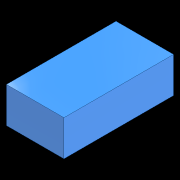
# Autodesk Inventor part: 2s 250mAh Mockup
Saved by Autodesk Inventor 2022 (Build 260153000, 153)
## iProperties
Created: 2022-09-18
Part Number: 2s 250mAh Mockup
Material: Generic
Document SubType Name: Modeling
Designer: tandu
Density: 1.4652 g/cm^3
Appearance: Cyan
Mass: 16 g
Surface Area: 32.66 cm^2
Volume: 10.92 cm^3
Author: tandu
Autodesk Inventor part; units mm, degrees
ref_plane "YZ Plane" through (0, 0, 0) normal (1, 0, 0) x (0, 1, 0)
ref_plane "XZ Plane" through (0, 0, 0) normal (0, 1, 0) x (-1, 0, 0)
ref_plane "XY Plane" through (0, 0, 0) normal (0, 0, 1) x (1, 0, 0)
sketch "Sketch1" plane through (0, 0, 0) normal (0, 1, 0) x (-1, 0, 0)
  line L0 (0, 0) -> (21, 0)
  line L1 (21, 0) -> (21, -40)
  line L2 (21, -40) -> (0, -40)
  line L3 (0, -40) -> (0, 0)
  dimension "d0" = 21
  dimension "d1" = 40
  constraints: 8 end point, 2 parallel, 1 horizontal, 1 perpendicular
  measures "d0" distance of L1.end L2.end
  measures "d1" distance of L0.end L1.end
extrude "Extrusion1" add sketch "Sketch1" along normal blind 13
body "Solid1"
